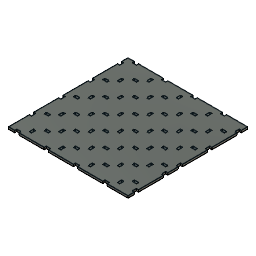
echiquier bas (Autodesk Fusion 360 design; units mm, degrees)
part number: 2026-06-29-10-21-54-786
Autodesk Fusion 360 part; units mm, degrees
sketch "Esquisse1" plane through (0, 0, 0) normal (0, 0, 1) x (1, 0, 0)
  line L0 (0, 0) -> (5, 0)
  line L1 (5, 0) -> (5, 35)
  line L2 (5, 35) -> (0, 35)
  line L3 (0, 35) -> (0, 0)
  line L4 (0, 0) -> (35, 0)
  line L5 (35, 0) -> (35, 5)
  line L6 (35, 5) -> (0, 5)
  line L7 (0, 5) -> (0, 0)
  line L8 (0, 0) -> (35, 0)
  line L9 (35, 0) -> (35, 35)
  line L10 (35, 35) -> (0, 35)
  line L11 (0, 35) -> (0, 0)
  line L12 (15, 0) -> (25, 0)
  line L13 (25, 0) -> (25, 5)
  line L14 (25, 5) -> (15, 5)
  line L15 (15, 5) -> (15, 0)
  line L16 (0, 25) -> (5, 25)
  line L17 (5, 25) -> (5, 15)
  line L18 (5, 15) -> (0, 15)
  line L19 (0, 15) -> (0, 25)
  line L20 (35, 15) -> (35, 25)
  line L21 (35, 25) -> (40, 25)
  line L22 (40, 25) -> (40, 15)
  line L23 (40, 15) -> (35, 15)
  line L24 (85, 0) -> (95, 0)
  line L25 (85, 5) -> (85, 0)
  line L26 (95, 5) -> (85, 5)
  line L27 (95, 0) -> (95, 5)
  line L28 (105, 15) -> (105, 25)
  line L29 (105, 25) -> (110, 25)
  line L30 (110, 25) -> (110, 15)
  line L31 (110, 15) -> (105, 15)
  line L32 (155, 0) -> (165, 0)
  line L33 (155, 5) -> (155, 0)
  line L34 (165, 5) -> (155, 5)
  line L35 (165, 0) -> (165, 5)
  line L36 (175, 15) -> (175, 25)
  line L37 (175, 25) -> (180, 25)
  line L38 (180, 25) -> (180, 15)
  line L39 (180, 15) -> (175, 15)
  line L40 (225, 0) -> (235, 0)
  line L41 (225, 5) -> (225, 0)
  line L42 (235, 5) -> (225, 5)
  line L43 (235, 0) -> (235, 5)
  line L44 (245, 15) -> (245, 25)
  line L45 (245, 25) -> (250, 25)
  line L46 (250, 25) -> (250, 15)
  line L47 (250, 15) -> (245, 15)
  line L48 (0, 50) -> (0, 60)
  line L49 (0, 60) -> (5, 60)
  line L50 (5, 60) -> (5, 50)
  line L51 (5, 50) -> (0, 50)
  line L52 (15, 35) -> (25, 35)
  line L53 (15, 40) -> (15, 35)
  line L54 (25, 40) -> (15, 40)
  line L55 (25, 35) -> (25, 40)
  line L56 (50, 35) -> (60, 35)
  line L57 (50, 40) -> (50, 35)
  line L58 (60, 40) -> (50, 40)
  line L59 (60, 35) -> (60, 40)
  line L60 (70, 50) -> (70, 60)
  line L61 (70, 60) -> (75, 60)
  line L62 (75, 60) -> (75, 50)
  line L63 (75, 50) -> (70, 50)
  line L64 (120, 35) -> (130, 35)
  line L65 (120, 40) -> (120, 35)
  line L66 (130, 40) -> (120, 40)
  line L67 (130, 35) -> (130, 40)
  line L68 (140, 50) -> (140, 60)
  line L69 (140, 60) -> (145, 60)
  line L70 (145, 60) -> (145, 50)
  line L71 (145, 50) -> (140, 50)
  line L72 (190, 35) -> (200, 35)
  line L73 (190, 40) -> (190, 35)
  line L74 (200, 40) -> (190, 40)
  line L75 (200, 35) -> (200, 40)
  line L76 (210, 50) -> (210, 60)
  line L77 (210, 60) -> (215, 60)
  line L78 (215, 60) -> (215, 50)
  line L79 (215, 50) -> (210, 50)
  line L80 (260, 35) -> (270, 35)
  line L81 (260, 40) -> (260, 35)
  line L82 (270, 40) -> (260, 40)
  line L83 (270, 35) -> (270, 40)
  line L84 (280, 15) -> (280, 25)
  line L85 (280, 25) -> (285, 25)
  line L86 (285, 25) -> (285, 15)
  line L87 (285, 15) -> (280, 15)
  line L88 (280, 50) -> (280, 60)
  line L89 (280, 60) -> (285, 60)
  line L90 (285, 60) -> (285, 50)
  line L91 (285, 50) -> (280, 50)
  line L92 (140, 120) -> (140, 130)
  line L93 (70, 120) -> (70, 130)
  line L94 (165, 70) -> (165, 75)
  line L95 (70, 130) -> (75, 130)
  line L96 (105, 95) -> (110, 95)
  line L97 (175, 95) -> (180, 95)
  line L98 (235, 70) -> (235, 75)
  line L99 (270, 110) -> (260, 110)
  line L100 (155, 70) -> (165, 70)
  line L101 (145, 130) -> (145, 120)
  line L102 (120, 110) -> (120, 105)
  line L103 (285, 85) -> (280, 85)
  line L104 (285, 120) -> (280, 120)
  line L105 (75, 120) -> (70, 120)
  line L106 (50, 105) -> (60, 105)
  line L107 (110, 85) -> (105, 85)
  line L108 (60, 110) -> (50, 110)
  line L109 (210, 120) -> (210, 130)
  line L110 (200, 105) -> (200, 110)
  line L111 (75, 130) -> (75, 120)
  line L112 (225, 70) -> (235, 70)
  line L113 (210, 130) -> (215, 130)
  line L114 (270, 105) -> (270, 110)
  line L115 (130, 110) -> (120, 110)
  line L116 (235, 75) -> (225, 75)
  line L117 (245, 85) -> (245, 95)
  line L118 (60, 105) -> (60, 110)
  line L119 (110, 95) -> (110, 85)
  line L120 (190, 110) -> (190, 105)
  line L121 (130, 105) -> (130, 110)
  line L122 (105, 85) -> (105, 95)
  line L123 (120, 105) -> (130, 105)
  line L124 (250, 85) -> (245, 85)
  line L125 (215, 130) -> (215, 120)
  line L126 (280, 95) -> (285, 95)
  line L127 (260, 110) -> (260, 105)
  line L128 (50, 110) -> (50, 105)
  line L129 (85, 75) -> (85, 70)
  line L130 (280, 120) -> (280, 130)
  line L131 (245, 95) -> (250, 95)
  line L132 (225, 75) -> (225, 70)
  line L133 (285, 95) -> (285, 85)
  line L134 (280, 130) -> (285, 130)
  line L135 (260, 105) -> (270, 105)
  line L136 (280, 85) -> (280, 95)
  line L137 (200, 110) -> (190, 110)
  line L138 (190, 105) -> (200, 105)
  line L139 (145, 120) -> (140, 120)
  line L140 (140, 130) -> (145, 130)
  line L141 (95, 75) -> (85, 75)
  line L142 (250, 95) -> (250, 85)
  line L143 (180, 85) -> (175, 85)
  line L144 (85, 70) -> (95, 70)
  line L145 (215, 120) -> (210, 120)
  line L146 (155, 75) -> (155, 70)
  line L147 (180, 95) -> (180, 85)
  line L148 (175, 85) -> (175, 95)
  line L149 (285, 130) -> (285, 120)
  line L150 (165, 75) -> (155, 75)
  line L151 (95, 70) -> (95, 75)
  line L152 (35, 95) -> (40, 95)
  line L153 (40, 95) -> (40, 85)
  line L154 (40, 85) -> (35, 85)
  line L155 (35, 70) -> (35, 105)
  line L156 (0, 70) -> (35, 70)
  line L157 (35, 75) -> (0, 75)
  line L158 (15, 75) -> (15, 70)
  line L159 (25, 70) -> (25, 75)
  line L160 (140, 190) -> (140, 200)
  line L161 (70, 190) -> (70, 200)
  line L162 (165, 140) -> (165, 145)
  line L163 (70, 200) -> (75, 200)
  line L164 (105, 165) -> (110, 165)
  line L165 (175, 165) -> (180, 165)
  line L166 (235, 140) -> (235, 145)
  line L167 (270, 180) -> (260, 180)
  line L168 (155, 140) -> (165, 140)
  line L169 (145, 200) -> (145, 190)
  line L170 (120, 180) -> (120, 175)
  line L171 (285, 155) -> (280, 155)
  line L172 (285, 190) -> (280, 190)
  line L173 (75, 190) -> (70, 190)
  line L174 (50, 175) -> (60, 175)
  line L175 (110, 155) -> (105, 155)
  line L176 (60, 180) -> (50, 180)
  line L177 (210, 190) -> (210, 200)
  line L178 (200, 175) -> (200, 180)
  line L179 (75, 200) -> (75, 190)
  line L180 (225, 140) -> (235, 140)
  line L181 (210, 200) -> (215, 200)
  line L182 (270, 175) -> (270, 180)
  line L183 (130, 180) -> (120, 180)
  line L184 (235, 145) -> (225, 145)
  line L185 (245, 155) -> (245, 165)
  line L186 (60, 175) -> (60, 180)
  line L187 (110, 165) -> (110, 155)
  line L188 (190, 180) -> (190, 175)
  line L189 (130, 175) -> (130, 180)
  line L190 (105, 155) -> (105, 165)
  line L191 (120, 175) -> (130, 175)
  line L192 (250, 155) -> (245, 155)
  line L193 (215, 200) -> (215, 190)
  line L194 (280, 165) -> (285, 165)
  line L195 (260, 180) -> (260, 175)
  line L196 (50, 180) -> (50, 175)
  line L197 (85, 145) -> (85, 140)
  line L198 (280, 190) -> (280, 200)
  line L199 (245, 165) -> (250, 165)
  line L200 (225, 145) -> (225, 140)
  line L201 (285, 165) -> (285, 155)
  line L202 (280, 200) -> (285, 200)
  line L203 (260, 175) -> (270, 175)
  line L204 (280, 155) -> (280, 165)
  line L205 (200, 180) -> (190, 180)
  line L206 (190, 175) -> (200, 175)
  line L207 (145, 190) -> (140, 190)
  line L208 (140, 200) -> (145, 200)
  line L209 (95, 145) -> (85, 145)
  line L210 (250, 165) -> (250, 155)
  line L211 (180, 155) -> (175, 155)
  line L212 (85, 140) -> (95, 140)
  line L213 (215, 190) -> (210, 190)
  line L214 (155, 145) -> (155, 140)
  line L215 (180, 165) -> (180, 155)
  line L216 (175, 155) -> (175, 165)
  line L217 (285, 200) -> (285, 190)
  line L218 (165, 145) -> (155, 145)
  line L219 (95, 140) -> (95, 145)
  line L220 (35, 165) -> (40, 165)
  line L221 (40, 165) -> (40, 155)
  line L222 (40, 155) -> (35, 155)
  line L223 (35, 140) -> (35, 175)
  line L224 (0, 140) -> (35, 140)
  line L225 (35, 145) -> (0, 145)
  line L226 (15, 145) -> (15, 140)
  line L227 (25, 140) -> (25, 145)
  line L228 (140, 260) -> (140, 270)
  line L229 (70, 260) -> (70, 270)
  line L230 (165, 210) -> (165, 215)
  line L231 (70, 270) -> (75, 270)
  line L232 (105, 235) -> (110, 235)
  line L233 (175, 235) -> (180, 235)
  line L234 (235, 210) -> (235, 215)
  line L235 (270, 250) -> (260, 250)
  line L236 (155, 210) -> (165, 210)
  line L237 (145, 270) -> (145, 260)
  line L238 (120, 250) -> (120, 245)
  line L239 (285, 225) -> (280, 225)
  line L240 (285, 260) -> (280, 260)
  line L241 (75, 260) -> (70, 260)
  line L242 (50, 245) -> (60, 245)
  line L243 (110, 225) -> (105, 225)
  line L244 (60, 250) -> (50, 250)
  line L245 (210, 260) -> (210, 270)
  line L246 (200, 245) -> (200, 250)
  line L247 (75, 270) -> (75, 260)
  line L248 (225, 210) -> (235, 210)
  line L249 (210, 270) -> (215, 270)
  line L250 (270, 245) -> (270, 250)
  line L251 (130, 250) -> (120, 250)
  line L252 (235, 215) -> (225, 215)
  line L253 (245, 225) -> (245, 235)
  line L254 (60, 245) -> (60, 250)
  line L255 (110, 235) -> (110, 225)
  line L256 (190, 250) -> (190, 245)
  line L257 (130, 245) -> (130, 250)
  line L258 (105, 225) -> (105, 235)
  line L259 (120, 245) -> (130, 245)
  line L260 (250, 225) -> (245, 225)
  line L261 (215, 270) -> (215, 260)
  line L262 (280, 235) -> (285, 235)
  line L263 (260, 250) -> (260, 245)
  line L264 (50, 250) -> (50, 245)
  line L265 (85, 215) -> (85, 210)
  line L266 (280, 260) -> (280, 270)
  line L267 (245, 235) -> (250, 235)
  line L268 (225, 215) -> (225, 210)
  line L269 (285, 235) -> (285, 225)
  line L270 (280, 270) -> (285, 270)
  line L271 (260, 245) -> (270, 245)
  line L272 (280, 225) -> (280, 235)
  line L273 (200, 250) -> (190, 250)
  line L274 (190, 245) -> (200, 245)
  line L275 (145, 260) -> (140, 260)
  line L276 (140, 270) -> (145, 270)
  line L277 (95, 215) -> (85, 215)
  line L278 (250, 235) -> (250, 225)
  line L279 (180, 225) -> (175, 225)
  line L280 (85, 210) -> (95, 210)
  line L281 (215, 260) -> (210, 260)
  line L282 (155, 215) -> (155, 210)
  line L283 (180, 235) -> (180, 225)
  line L284 (175, 225) -> (175, 235)
  line L285 (285, 270) -> (285, 260)
  line L286 (165, 215) -> (155, 215)
  line L287 (95, 210) -> (95, 215)
  line L288 (35, 235) -> (40, 235)
  line L289 (40, 235) -> (40, 225)
  line L290 (40, 225) -> (35, 225)
  line L291 (35, 210) -> (35, 245)
  line L292 (0, 210) -> (35, 210)
  line L293 (35, 215) -> (0, 215)
  line L294 (15, 215) -> (15, 210)
  line L295 (25, 210) -> (25, 215)
  line L296 (140, 330) -> (140, 340)
  line L297 (70, 330) -> (70, 340)
  line L298 (165, 280) -> (165, 285)
  line L299 (70, 340) -> (75, 340)
  line L300 (105, 305) -> (110, 305)
  line L301 (175, 305) -> (180, 305)
  line L302 (235, 280) -> (235, 285)
  line L303 (270, 320) -> (260, 320)
  line L304 (155, 280) -> (165, 280)
  line L305 (145, 340) -> (145, 330)
  line L306 (120, 320) -> (120, 315)
  line L307 (285, 295) -> (280, 295)
  line L308 (285, 330) -> (280, 330)
  line L309 (75, 330) -> (70, 330)
  line L310 (50, 315) -> (60, 315)
  line L311 (110, 295) -> (105, 295)
  line L312 (210, 330) -> (210, 340)
  line L313 (200, 315) -> (200, 320)
  line L314 (75, 340) -> (75, 330)
  line L315 (225, 280) -> (235, 280)
  line L316 (210, 340) -> (215, 340)
  line L317 (270, 315) -> (270, 320)
  line L318 (130, 320) -> (120, 320)
  line L319 (235, 285) -> (225, 285)
  line L320 (245, 295) -> (245, 305)
  line L321 (60, 315) -> (60, 320)
  line L322 (110, 305) -> (110, 295)
  line L323 (190, 320) -> (190, 315)
  line L324 (130, 315) -> (130, 320)
  line L325 (105, 295) -> (105, 305)
  line L326 (120, 315) -> (130, 315)
  line L327 (250, 295) -> (245, 295)
  line L328 (215, 340) -> (215, 330)
  line L329 (280, 305) -> (285, 305)
  line L330 (260, 320) -> (260, 315)
  line L331 (85, 285) -> (85, 280)
  line L332 (280, 330) -> (280, 340)
  line L333 (245, 305) -> (250, 305)
  line L334 (225, 285) -> (225, 280)
  line L335 (285, 305) -> (285, 295)
  line L336 (280, 340) -> (285, 340)
  line L337 (260, 315) -> (270, 315)
  line L338 (280, 295) -> (280, 305)
  line L339 (200, 320) -> (190, 320)
  line L340 (190, 315) -> (200, 315)
  line L341 (145, 330) -> (140, 330)
  line L342 (140, 340) -> (145, 340)
  line L343 (95, 285) -> (85, 285)
  line L344 (250, 305) -> (250, 295)
  line L345 (180, 295) -> (175, 295)
  line L346 (85, 280) -> (95, 280)
  line L347 (215, 330) -> (210, 330)
  line L348 (155, 285) -> (155, 280)
  line L349 (180, 305) -> (180, 295)
  line L350 (175, 295) -> (175, 305)
  line L351 (285, 340) -> (285, 330)
  line L352 (165, 285) -> (155, 285)
  line L353 (95, 280) -> (95, 285)
  line L354 (35, 305) -> (40, 305)
  line L355 (40, 305) -> (40, 295)
  line L356 (40, 295) -> (35, 295)
  line L357 (35, 280) -> (35, 315)
  line L358 (0, 280) -> (35, 280)
  line L359 (35, 285) -> (0, 285)
  line L360 (15, 285) -> (15, 280)
  line L361 (25, 280) -> (25, 285)
  line L362 (0, 0) -> (285, 0)
  line L363 (285, 0) -> (285, 285)
  line L364 (285, 285) -> (0, 285)
  line L365 (0, 285) -> (0, 0)
  line L366 (5, 130) -> (5, 120)
  line L367 (0, 130) -> (5, 130)
  line L368 (5, 120) -> (0, 120)
  line L369 (5, 200) -> (5, 190)
  line L370 (0, 200) -> (5, 200)
  line L371 (5, 190) -> (0, 190)
  line L372 (5, 270) -> (5, 260)
  line L373 (0, 270) -> (5, 270)
  line L374 (5, 260) -> (0, 260)
  dimension "d9" = 5
  dimension "d10" = 5
  dimension "d11" = 35
  dimension "d12" = 35
  dimension "d13" = 10
  dimension "d14" = 10
  dimension "d15" = 10
  dimension "d16" = 10
  dimension "d19" = 35
  dimension "d20" = 35
  dimension "d34" = 285
  constraint horizontal L0
  constraint vertical L1
  constraint horizontal L2
  constraint vertical L3
  constraint coincident L0.start L3.end
  constraint horizontal L4
  constraint vertical L5
  constraint horizontal L6
  constraint vertical L7
  constraint horizontal L8
  constraint vertical L9
  constraint horizontal L10
  constraint vertical L11
  constraint collinear L5 L9
  constraint collinear L2 L10
  constraint horizontal L12
  constraint vertical L13
  constraint horizontal L14
  constraint vertical L15
  constraint coincident L6 L13.end
  constraint coincident L4 L12.start
  constraint horizontal L16
  constraint vertical L17
  constraint horizontal L18
  constraint vertical L19
  constraint coincident L1 L17.end
  constraint coincident L11 L16.start
  constraint horizontal L362
  constraint vertical L363
  constraint horizontal L364
  constraint vertical L365
  measures "d9" distance of L1 L3
  measures "d10" distance of L4 L6
  measures "d11" distance of L8 L10
  measures "d12" distance of L9 L11
  measures "d13" distance of L1 L15
  measures "d14" distance of L9 L13
  measures "d15" distance of L6 L18
  measures "d16" distance of L10 L16
  measures "d34" distance of L0.start L359.end
extrude "Extrusion1" add sketch "Esquisse1" along normal blind 5 contours L0 L1 L3 L4 L6 L7 L8 L11 L362 L365 | L1 L4 L6 L8 L15 L362 | L1 L3 L6 L11 L18 L365 | L1 L6 L9 L10 L14 L17 L20 L52 | L1 L3 L11 L16 L17 L18 L19 L365 | L4 L5 L6 L8 L9 L13 L362 | L1 L2 L3 L10 L11 L16 L365 | L2 L5 L9 L10 L21 L22 L23 L25 L26 L27 L33 L34 L35 L41 L42 L43 L49 L50 L51 L53 L54 L55 L84 L85 L87 L88 L89 L91 L103 L104 L126 L130 L134 L136 L155 L156 L157 L171 L172 L194 L198 L202 L204 L223 L224 L225 L239 L240 L262 L266 L270 L272 L291 L292 L293 L298 L302 L304 L315 L331 L334 L346 L348 L353 L357 L358 L362 L363 L364 L365 L366 L367 L368 L369 L370 L371 L372 L373 L374 | L10 L52 L53 L54 L55 | L156 L157 L158 L365 | L155 L156 L157 L159 | L224 L225 L226 L365 | L223 L224 L225 L227 | L88 L89 L90 L91 L363 | L292 L293 L294 L365 | L291 L292 L293 L295 | L358 L359 L360 L364 L365 | L171 L194 L201 L204 L363 | L357 L358 L359 L361 L364 | L239 L262 L269 L272 L363
sketch "Esquisse2" plane through (0, 0, 5) normal (0, 0, 1) x (-1, 0, 0)
  line L0 (-270, -105) -> (-260, -105)
  line L1 (-260, -105) -> (-260, -110)
  line L2 (-260, -110) -> (-270, -110)
  line L3 (-270, -110) -> (-270, -105)
  line L4 (-270, -40) -> (-270, -35)
  line L5 (-270, -35) -> (-260, -35)
  line L6 (-260, -35) -> (-260, -40)
  line L7 (-260, -40) -> (-270, -40)
  line L8 (-95, -145) -> (-95, -140)
  line L9 (-95, -140) -> (-85, -140)
  line L10 (-85, -140) -> (-85, -145)
  line L11 (-85, -145) -> (-95, -145)
  line L12 (-50, -105) -> (-50, -110)
  line L13 (-50, -110) -> (-60, -110)
  line L14 (-60, -110) -> (-60, -105)
  line L15 (-60, -105) -> (-50, -105)
  line L16 (-245, -95) -> (-250, -95)
  line L17 (-250, -95) -> (-250, -85)
  line L18 (-250, -85) -> (-245, -85)
  line L19 (-245, -85) -> (-245, -95)
  line L20 (-110, -155) -> (-105, -155)
  line L21 (-105, -155) -> (-105, -165)
  line L22 (-105, -165) -> (-110, -165)
  line L23 (-110, -165) -> (-110, -155)
  line L24 (-130, -105) -> (-120, -105)
  line L25 (-120, -105) -> (-120, -110)
  line L26 (-120, -110) -> (-130, -110)
  line L27 (-130, -110) -> (-130, -105)
  line L28 (-70, -270) -> (-75, -270)
  line L29 (-75, -270) -> (-75, -260)
  line L30 (-75, -260) -> (-70, -260)
  line L31 (-70, -260) -> (-70, -270)
  line L32 (-200, -40) -> (-200, -35)
  line L33 (-200, -35) -> (-190, -35)
  line L34 (-190, -35) -> (-190, -40)
  line L35 (-190, -40) -> (-200, -40)
  line L36 (-130, -245) -> (-120, -245)
  line L37 (-120, -245) -> (-120, -250)
  line L38 (-120, -250) -> (-130, -250)
  line L39 (-130, -250) -> (-130, -245)
  line L40 (-270, -245) -> (-260, -245)
  line L41 (-260, -245) -> (-260, -250)
  line L42 (-260, -250) -> (-270, -250)
  line L43 (-270, -250) -> (-270, -245)
  line L44 (-70, -130) -> (-75, -130)
  line L45 (-75, -130) -> (-75, -120)
  line L46 (-75, -120) -> (-70, -120)
  line L47 (-70, -120) -> (-70, -130)
  line L48 (-200, -105) -> (-190, -105)
  line L49 (-190, -105) -> (-190, -110)
  line L50 (-190, -110) -> (-200, -110)
  line L51 (-200, -110) -> (-200, -105)
  line L52 (-245, -165) -> (-250, -165)
  line L53 (-250, -165) -> (-250, -155)
  line L54 (-250, -155) -> (-245, -155)
  line L55 (-245, -155) -> (-245, -165)
  line L56 (-145, -60) -> (-145, -50)
  line L57 (-145, -50) -> (-140, -50)
  line L58 (-140, -50) -> (-140, -60)
  line L59 (-140, -60) -> (-145, -60)
  line L60 (-200, -175) -> (-190, -175)
  line L61 (-190, -175) -> (-190, -180)
  line L62 (-190, -180) -> (-200, -180)
  line L63 (-200, -180) -> (-200, -175)
  line L64 (-140, -190) -> (-140, -200)
  line L65 (-140, -200) -> (-145, -200)
  line L66 (-145, -200) -> (-145, -190)
  line L67 (-145, -190) -> (-140, -190)
  line L68 (-130, -40) -> (-130, -35)
  line L69 (-130, -35) -> (-120, -35)
  line L70 (-120, -35) -> (-120, -40)
  line L71 (-120, -40) -> (-130, -40)
  line L72 (-40, -235) -> (-40, -225)
  line L73 (-40, -225) -> (-35, -225)
  line L74 (-35, -225) -> (-35, -235)
  line L75 (-35, -235) -> (-40, -235)
  line L76 (-155, -75) -> (-165, -75)
  line L77 (-165, -75) -> (-165, -70)
  line L78 (-165, -70) -> (-155, -70)
  line L79 (-155, -70) -> (-155, -75)
  line L80 (-40, -165) -> (-40, -155)
  line L81 (-40, -155) -> (-35, -155)
  line L82 (-35, -155) -> (-35, -165)
  line L83 (-35, -165) -> (-40, -165)
  line L84 (-215, -200) -> (-215, -190)
  line L85 (-215, -190) -> (-210, -190)
  line L86 (-210, -190) -> (-210, -200)
  line L87 (-210, -200) -> (-215, -200)
  line L88 (-110, -25) -> (-110, -15)
  line L89 (-110, -15) -> (-105, -15)
  line L90 (-105, -15) -> (-105, -25)
  line L91 (-105, -25) -> (-110, -25)
  line L92 (-155, -145) -> (-165, -145)
  line L93 (-165, -145) -> (-165, -140)
  line L94 (-165, -140) -> (-155, -140)
  line L95 (-155, -140) -> (-155, -145)
  line L96 (-15, -285) -> (0, -285)
  line L97 (0, -285) -> (0, -270)
  line L98 (0, -270) -> (-5, -270)
  line L99 (-5, -270) -> (-5, -260)
  line L100 (-5, -260) -> (0, -260)
  line L101 (0, -260) -> (0, -200)
  line L102 (0, -200) -> (-5, -200)
  line L103 (-5, -200) -> (-5, -190)
  line L104 (-5, -190) -> (0, -190)
  line L105 (0, -190) -> (0, -130)
  line L106 (0, -130) -> (-5, -130)
  line L107 (-5, -130) -> (-5, -120)
  line L108 (-5, -120) -> (0, -120)
  line L109 (0, -120) -> (0, -60)
  line L110 (0, -60) -> (-5, -60)
  line L111 (-5, -60) -> (-5, -50)
  line L112 (-5, -50) -> (0, -50)
  line L113 (0, -50) -> (0, 0)
  line L114 (0, 0) -> (-15, 0)
  line L115 (-15, 0) -> (-15, -5)
  line L116 (-15, -5) -> (-25, -5)
  line L117 (-25, -5) -> (-25, 0)
  line L118 (-25, 0) -> (-85, 0)
  line L119 (-85, 0) -> (-85, -5)
  line L120 (-85, -5) -> (-95, -5)
  line L121 (-95, -5) -> (-95, 0)
  line L122 (-95, 0) -> (-155, 0)
  line L123 (-155, 0) -> (-155, -5)
  line L124 (-155, -5) -> (-165, -5)
  line L125 (-165, -5) -> (-165, 0)
  line L126 (-165, 0) -> (-225, 0)
  line L127 (-225, 0) -> (-225, -5)
  line L128 (-225, -5) -> (-235, -5)
  line L129 (-235, -5) -> (-235, 0)
  line L130 (-235, 0) -> (-285, 0)
  line L131 (-285, 0) -> (-285, -15)
  line L132 (-285, -15) -> (-280, -15)
  line L133 (-280, -15) -> (-280, -25)
  line L134 (-280, -25) -> (-285, -25)
  line L135 (-285, -25) -> (-285, -85)
  line L136 (-285, -85) -> (-280, -85)
  line L137 (-280, -85) -> (-280, -95)
  line L138 (-280, -95) -> (-285, -95)
  line L139 (-285, -95) -> (-285, -120)
  line L140 (-285, -120) -> (-280, -120)
  line L141 (-280, -120) -> (-280, -130)
  line L142 (-280, -130) -> (-285, -130)
  line L143 (-285, -130) -> (-285, -190)
  line L144 (-285, -190) -> (-280, -190)
  line L145 (-280, -190) -> (-280, -200)
  line L146 (-280, -200) -> (-285, -200)
  line L147 (-285, -200) -> (-285, -260)
  line L148 (-285, -260) -> (-280, -260)
  line L149 (-280, -260) -> (-280, -270)
  line L150 (-280, -270) -> (-285, -270)
  line L151 (-285, -270) -> (-285, -285)
  line L152 (-285, -285) -> (-235, -285)
  line L153 (-235, -285) -> (-235, -280)
  line L154 (-235, -280) -> (-225, -280)
  line L155 (-225, -280) -> (-225, -285)
  line L156 (-225, -285) -> (-165, -285)
  line L157 (-165, -285) -> (-165, -280)
  line L158 (-165, -280) -> (-155, -280)
  line L159 (-155, -280) -> (-155, -285)
  line L160 (-155, -285) -> (-95, -285)
  line L161 (-95, -285) -> (-95, -280)
  line L162 (-95, -280) -> (-85, -280)
  line L163 (-85, -280) -> (-85, -285)
  line L164 (-85, -285) -> (-25, -285)
  line L165 (-25, -285) -> (-25, -280)
  line L166 (-25, -280) -> (-15, -280)
  line L167 (-15, -280) -> (-15, -285)
  line L168 (-25, -215) -> (-25, -210)
  line L169 (-25, -210) -> (-15, -210)
  line L170 (-15, -210) -> (-15, -215)
  line L171 (-15, -215) -> (-25, -215)
  line L172 (-40, -25) -> (-40, -15)
  line L173 (-40, -15) -> (-35, -15)
  line L174 (-35, -15) -> (-35, -25)
  line L175 (-35, -25) -> (-40, -25)
  line L176 (-25, -145) -> (-25, -140)
  line L177 (-25, -140) -> (-15, -140)
  line L178 (-15, -140) -> (-15, -145)
  line L179 (-15, -145) -> (-25, -145)
  line L180 (-25, -75) -> (-25, -70)
  line L181 (-25, -70) -> (-15, -70)
  line L182 (-15, -70) -> (-15, -75)
  line L183 (-15, -75) -> (-25, -75)
  line L184 (-140, -260) -> (-140, -270)
  line L185 (-140, -270) -> (-145, -270)
  line L186 (-145, -270) -> (-145, -260)
  line L187 (-145, -260) -> (-140, -260)
  line L188 (-200, -245) -> (-190, -245)
  line L189 (-190, -245) -> (-190, -250)
  line L190 (-190, -250) -> (-200, -250)
  line L191 (-200, -250) -> (-200, -245)
  line L192 (-50, -245) -> (-50, -250)
  line L193 (-50, -250) -> (-60, -250)
  line L194 (-60, -250) -> (-60, -245)
  line L195 (-60, -245) -> (-50, -245)
  line L196 (-180, -225) -> (-175, -225)
  line L197 (-175, -225) -> (-175, -235)
  line L198 (-175, -235) -> (-180, -235)
  line L199 (-180, -235) -> (-180, -225)
  line L200 (-270, -175) -> (-260, -175)
  line L201 (-260, -175) -> (-260, -180)
  line L202 (-260, -180) -> (-270, -180)
  line L203 (-270, -180) -> (-270, -175)
  line L204 (-225, -140) -> (-225, -145)
  line L205 (-225, -145) -> (-235, -145)
  line L206 (-235, -145) -> (-235, -140)
  line L207 (-235, -140) -> (-225, -140)
  line L208 (-155, -215) -> (-165, -215)
  line L209 (-165, -215) -> (-165, -210)
  line L210 (-165, -210) -> (-155, -210)
  line L211 (-155, -210) -> (-155, -215)
  line L212 (-60, -40) -> (-60, -35)
  line L213 (-60, -35) -> (-50, -35)
  line L214 (-50, -35) -> (-50, -40)
  line L215 (-50, -40) -> (-60, -40)
  line L216 (-180, -155) -> (-175, -155)
  line L217 (-175, -155) -> (-175, -165)
  line L218 (-175, -165) -> (-180, -165)
  line L219 (-180, -165) -> (-180, -155)
  line L220 (-140, -120) -> (-140, -130)
  line L221 (-140, -130) -> (-145, -130)
  line L222 (-145, -130) -> (-145, -120)
  line L223 (-145, -120) -> (-140, -120)
  line L224 (-180, -25) -> (-180, -15)
  line L225 (-180, -15) -> (-175, -15)
  line L226 (-175, -15) -> (-175, -25)
  line L227 (-175, -25) -> (-180, -25)
  line L228 (-180, -85) -> (-175, -85)
  line L229 (-175, -85) -> (-175, -95)
  line L230 (-175, -95) -> (-180, -95)
  line L231 (-180, -95) -> (-180, -85)
  line L232 (-250, -25) -> (-250, -15)
  line L233 (-250, -15) -> (-245, -15)
  line L234 (-245, -15) -> (-245, -25)
  line L235 (-245, -25) -> (-250, -25)
  line L236 (-110, -225) -> (-105, -225)
  line L237 (-105, -225) -> (-105, -235)
  line L238 (-105, -235) -> (-110, -235)
  line L239 (-110, -235) -> (-110, -225)
  line L240 (-130, -175) -> (-120, -175)
  line L241 (-120, -175) -> (-120, -180)
  line L242 (-120, -180) -> (-130, -180)
  line L243 (-130, -180) -> (-130, -175)
  line L244 (-215, -130) -> (-215, -120)
  line L245 (-215, -120) -> (-210, -120)
  line L246 (-210, -120) -> (-210, -130)
  line L247 (-210, -130) -> (-215, -130)
  line L248 (-110, -85) -> (-105, -85)
  line L249 (-105, -85) -> (-105, -95)
  line L250 (-105, -95) -> (-110, -95)
  line L251 (-110, -95) -> (-110, -85)
  line L252 (-225, -70) -> (-225, -75)
  line L253 (-225, -75) -> (-235, -75)
  line L254 (-235, -75) -> (-235, -70)
  line L255 (-235, -70) -> (-225, -70)
  line L256 (-215, -60) -> (-215, -50)
  line L257 (-215, -50) -> (-210, -50)
  line L258 (-210, -50) -> (-210, -60)
  line L259 (-210, -60) -> (-215, -60)
  line L260 (-245, -235) -> (-250, -235)
  line L261 (-250, -235) -> (-250, -225)
  line L262 (-250, -225) -> (-245, -225)
  line L263 (-245, -225) -> (-245, -235)
  line L264 (-95, -75) -> (-95, -70)
  line L265 (-95, -70) -> (-85, -70)
  line L266 (-85, -70) -> (-85, -75)
  line L267 (-85, -75) -> (-95, -75)
  line L268 (-215, -270) -> (-215, -260)
  line L269 (-215, -260) -> (-210, -260)
  line L270 (-210, -260) -> (-210, -270)
  line L271 (-210, -270) -> (-215, -270)
  line L272 (-70, -200) -> (-75, -200)
  line L273 (-75, -200) -> (-75, -190)
  line L274 (-75, -190) -> (-70, -190)
  line L275 (-70, -190) -> (-70, -200)
  line L276 (-75, -60) -> (-75, -50)
  line L277 (-75, -50) -> (-70, -50)
  line L278 (-70, -50) -> (-70, -60)
  line L279 (-70, -60) -> (-75, -60)
  line L280 (-225, -210) -> (-225, -215)
  line L281 (-225, -215) -> (-235, -215)
  line L282 (-235, -215) -> (-235, -210)
  line L283 (-235, -210) -> (-225, -210)
  line L284 (-40, -95) -> (-40, -85)
  line L285 (-40, -85) -> (-35, -85)
  line L286 (-35, -85) -> (-35, -95)
  line L287 (-35, -95) -> (-40, -95)
  line L288 (-95, -215) -> (-95, -210)
  line L289 (-95, -210) -> (-85, -210)
  line L290 (-85, -210) -> (-85, -215)
  line L291 (-85, -215) -> (-95, -215)
  line L292 (-50, -175) -> (-50, -180)
  line L293 (-50, -180) -> (-60, -180)
  line L294 (-60, -180) -> (-60, -175)
  line L295 (-60, -175) -> (-50, -175)
